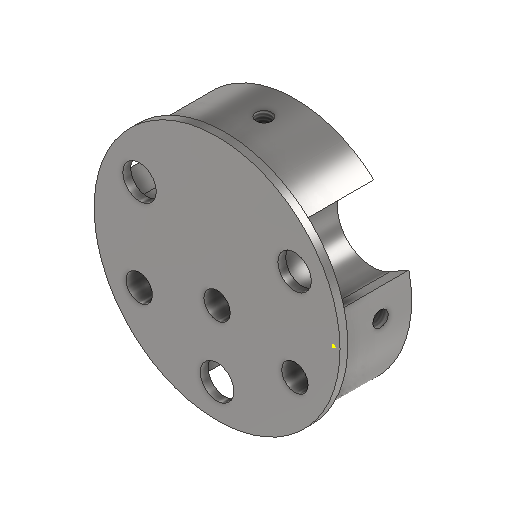
# Autodesk Inventor part: B_pipe_cylinder_5_1_1
Saved by Autodesk Inventor 2026.2 (Build 302298000, 298)
## iProperties
Created: 2026-02-02
Part Number: B_pipe_cylinder_5_1_1
Material: ステンレス鋼 440C
Document SubType Name: Modeling
Designer: zetsu
Density: 7.75 g/cm^3
Appearance: 半つや出し
Author: zetsu
Autodesk Inventor part; units mm, degrees
sketch "スケッチ2" plane through (0, 0, 0) normal (0, 0, 1) x (1, 0, 0)
  circle A0 centre (0, 0) radius 15.8
  dimension "d0" = 31.6
  constraints: 1 centre point, 1 coincident
  measures "d0" diameter of A0
extrude "押し出し1" add sketch "スケッチ2" against normal blind 10
sketch "スケッチ13" plane through (0, 0, 0) normal (0, 0, 1) x (1, 0, 0)
  circle A0 centre (0, -3) radius 1.7
  circle A1 centre (-10, -6) radius 1.7
  circle A2 centre (10, -6) radius 1.7
  line L0 (0, 0) -> (0, 17.9574) construction
  dimension "d90" = 3.4
  dimension "d91" = 3.4
  dimension "d92" = 3.4
  dimension "d93" = 3
  dimension "d94" = 6
  dimension "d95" = 10
  constraints: 3 centre point, 2 end point, 1 symmetric about line, 1 vertical
  measures "d90" diameter of A0
  measures "d91" diameter of A1
  measures "d92" diameter of A2
  measures "d93" distance of L0.start A0.centre
  measures "d94" vertical distance of A2.centre L0.start
  measures "d95" horizontal distance of A2.centre L0.start
extrude "押し出し11" cut sketch "スケッチ13" against normal through all
sketch "スケッチ14" plane through (0, 0, 0) normal (0, 0, 1) x (1, 0, 0)
  circle A0 centre (0, -11.5) radius 2.15
  circle A1 centre (9.9593, 5.75) radius 2.15
  circle A2 centre (-9.9593, 5.75) radius 2.15
  point P0 (0, 0)
  dimension "d98" = 4.3
  dimension "d99" = 11.5
  dimension "d102" = 360
  constraints: 3 centre point, 7 other
  measures "d98" diameter of A0
  measures "d99" distance of A0.centre point (0, 0)
extrude "押し出し12" cut sketch "スケッチ14" against normal blind 1
ref_plane "作業平面1" through (15, 0, 0) normal (1, 0, 0) x (0, 1, 0)
ref_plane "作業平面2" through (-15, 0, 0) normal (1, 0, 0) x (0, 1, 0)
ref_plane "作業平面3" through (0, 15, 0) normal (0, 1, 0) x (-1, 0, 0)
ref_plane "作業平面4" through (0, -15, 0) normal (0, 1, 0) x (-1, 0, 0)
sketch "スケッチ22" plane through (0, 0, -10) normal (0, 0, -1) x (-1, 0, 0)
  arc A0 (4.5, -11.5) -> (-4.5, -11.5) centre (0, -11.5) ccw
  line L0 (-4.5, -11.5) -> (-4.5, -15.8)
  line L1 (-4.5, -15.8) -> (4.5, -15.8)
  line L2 (4.5, -15.8) -> (4.5, -11.5)
  arc A1 (7.7093, 9.6471) -> (12.2093, 1.8529) centre (9.9593, 5.75) ccw
  line L3 (11.4332, 11.7971) -> (7.7093, 9.6471)
  line L4 (15.9332, 4.0029) -> (11.4332, 11.7971)
  line L5 (12.2093, 1.8529) -> (15.9332, 4.0029)
  arc A2 (-12.2093, 1.8529) -> (-7.7093, 9.6471) centre (-9.9593, 5.75) ccw
  line L6 (-15.9332, 4.0029) -> (-12.2093, 1.8529)
  line L7 (-11.4332, 11.7971) -> (-15.9332, 4.0029)
  line L8 (-7.7093, 9.6471) -> (-11.4332, 11.7971)
  point P0 (0, 0)
  dimension "d129" = 4.5
  dimension "d132" = 360
  constraints: 18 end point, 6 point on circle, 3 centre point, 2 perpendicular, 1 coincident, 1 vertical, 28 other
  measures "d129" radius of A0
extrude "押し出し17" cut sketch "スケッチ22" against normal blind 9
sketch "スケッチ23" plane through (15, 0, 0) normal (1, 0, 0) x (0, 1, 0)
  point P0 (0, 0)
sketch "スケッチ24" plane through (0, 0, -10) normal (0, 0, -1) x (-1, 0, 0)
  circle A0 centre (0, 0) radius 15.8
  circle A1 centre (0, 0) radius 15
  dimension "d136" = 30
  constraints: 2 centre point, 2 coincident
  measures "d136" diameter of A1
extrude "押し出し18" cut sketch "スケッチ24" against normal blind 9
sketch "スケッチ25" plane through (15, 0, 0) normal (1, 0, 0) x (0, 1, 0)
  circle A0 centre (0, -6) radius 1
  line L0 (-14.3091, -10) -> (3.2574, -10) projected
  line L1 (15.8, -1) -> (-15.8, -1) projected
  point P0 (0, 0)
  dimension "d139" = 2
  dimension "d141" = 5
  constraints: 1 centre point
  measures "d139" diameter of A0
  measures "d141" distance from line of A0.centre L1
sketch "スケッチ27" plane through (0, 15, 0) normal (0, 1, 0) x (-1, 0, 0)
  circle A0 centre (0, -6) radius 1
  line L0 (15.8, -1) -> (-15.8, -1) projected
  point P0 (0, 0)
  dimension "d142" = 2
  dimension "d143" = 5
  constraints: 1 centre point
  measures "d142" diameter of A0
  measures "d143" distance from line of L0 A0.centre
sketch "スケッチ28" plane through (-15, 0, 0) normal (1, 0, 0) x (0, 1, 0)
  circle A0 centre (0, -6) radius 1
  line L0 (15.8, -1) -> (-15.8, -1) projected
  point P0 (0, 0)
  dimension "d144" = 2
  dimension "d145" = 5
  constraints: 1 centre point
  measures "d144" diameter of A0
  measures "d145" distance from line of L0 A0.centre
extrude "押し出し19" cut sketch "スケッチ25" against normal blind 6
extrude "押し出し20" cut sketch "スケッチ27" against normal blind 6
extrude "押し出し21" cut sketch "スケッチ28" along normal blind 6
thread "ねじ9" size "M2x0.4" class "6H" standard "ANSI Metric M Profile" full length
thread "ねじ10" size "M2x0.4" class "6H" standard "ANSI Metric M Profile" full length
thread "ねじ11" size "M2x0.4" class "6H" standard "ANSI Metric M Profile" full length
